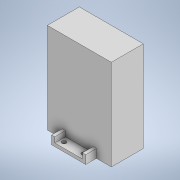
# Autodesk Inventor part: 80mm_テスト
Saved by Autodesk Inventor 2021.4 (Build 254397000, 397)
## iProperties
Created: 2023-06-14
Part Number: 80mm_テスト
Material: 一般
Document SubType Name: Modeling
Designer: Kota-M
Density: 1 g/cm^3
Appearance: 既定
Author: Kota-M
Autodesk Inventor part; units mm, degrees
ref_plane "YZ Plane" through (0, 0, 0) normal (1, 0, 0) x (0, 1, 0)
ref_plane "XZ Plane" through (0, 0, 0) normal (0, 1, 0) x (-1, 0, 0)
ref_plane "XY Plane" through (0, 0, 0) normal (0, 0, 1) x (1, 0, 0)
sketch "スケッチ1" plane through (0, 0, 0) normal (0, 1, 0) x (-1, 0, 0)
  line L0 (30, 15) -> (-30, 15)
  line L1 (-30, 15) -> (-30, -15)
  line L2 (-30, -15) -> (30, -15)
  line L3 (30, -15) -> (30, 15)
  line L4 (30, 15) -> (-30, -15) construction
  line L5 (-30, 15) -> (30, -15) construction
  point P0 (0, 0)
  dimension "d0" = 60
  dimension "d1" = 30
  constraints: 12 end point, 2 midpoint, 2 parallel, 1 horizontal, 1 perpendicular
  measures "d0" distance of L2.end L1.end
  measures "d1" distance of L1.end L0.end
extrude "押し出し1" add sketch "スケッチ1" along normal blind 85
sketch "スケッチ2" plane through (0, 0, 0) normal (0, -1, 0) x (1, 0, 0)
  line L0 (16, 5) -> (-16, 5)
  line L1 (-16, 5) -> (-16, 25)
  line L2 (-16, 25) -> (16, 25)
  line L3 (16, 25) -> (16, 5)
  line L4 (-30, 15) -> (30, 15) projected
  line L5 (16, 5) -> (-16, 25) construction
  line L6 (-16, 5) -> (16, 25) construction
  point P0 (0, 0)
  point P1 (0, 15)
  point P2 (-16, 15)
  point P3 (16, 15)
  dimension "d4" = 32
  dimension "d5" = 20
  constraints: 12 end point, 3 midpoint, 2 parallel, 1 horizontal, 1 perpendicular
  measures "d4" distance of L1.end L2.end
  measures "d5" distance of L0.end L1.end
extrude "押し出し2" add sketch "スケッチ2" against normal blind 3 contours L4 L1 L2 L3
sketch "スケッチ3" plane through (0, 3, 0) normal (0, 1, 0) x (1, 0, 0)
  line L0 (-16, -25) -> (16, -25) projected
  line L1 (-30, -15) -> (30, -15) projected
  line L2 (16, -25) -> (13, -25)
  line L3 (13, -25) -> (13, -15)
  line L4 (13, -15) -> (16, -15)
  line L5 (16, -15) -> (16, -25)
  line L6 (-16, -15) -> (-16, -25) projected
  line L7 (-16, -25) -> (-13, -25)
  line L8 (-13, -25) -> (-13, -15)
  line L9 (-13, -15) -> (-16, -15)
  line L10 (-16, -15) -> (-16, -25)
  point P0 (0, 0)
  point P1 (-13, -25)
  point P2 (-13, -15)
  point P3 (16, -15)
  dimension "d8" = 3
  dimension "d9" = 3
  constraints: 16 end point, 4 parallel, 2 horizontal, 2 perpendicular, 2 point on line
  measures "d8" distance of L3.end L4.end
  measures "d9" distance of L9.end L8.end
extrude "押し出し3" add sketch "スケッチ3" along normal blind 5 contours L6 L1 L8 L0 | L3 L1 L5 L0
sketch "スケッチ4" plane through (0, 3, 0) normal (0, 1, 0) x (1, 0, 0)
  line L0 (13, -25) -> (16, -25) projected
  line L1 (-13, -15) -> (-13, -25) projected
  line L2 (13, -25) -> (-13, -25)
  line L3 (-13, -25) -> (-13, -20)
  line L4 (-13, -20) -> (13, -20)
  line L5 (13, -20) -> (13, -25)
  line L6 (-13, -15) -> (13, -15) projected
  line L7 (9.3, -25) -> (-9.3, -25)
  line L8 (-9.3, -25) -> (-9.3, -15)
  line L9 (-9.3, -15) -> (9.3, -15)
  line L10 (9.3, -15) -> (9.3, -25)
  line L11 (9.3, -25) -> (-9.3, -15) construction
  line L12 (-9.3, -25) -> (9.3, -15) construction
  point P0 (0, 0)
  point P1 (0, -20)
  point P2 (9.3, -20)
  point P3 (-9.3, -20)
  dimension "d12" = 5
  dimension "d13" = 18.6
  constraints: 20 end point, 6 midpoint, 4 parallel, 2 horizontal, 2 perpendicular, 1 point on line
  measures "d12" distance between parallel lines of L4 L2
  measures "d13" distance of L8.end L9.end
hole "穴1" at (9.3, 3, 20) at (-9.3, 3, 20) direction (0, -1, 0) diameter 4 end through all
